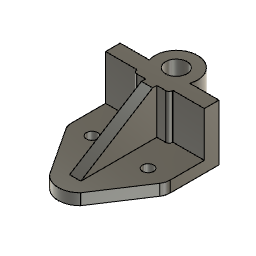
A3 (Autodesk Fusion 360 design; units mm, degrees)
Autodesk Fusion 360 part; units mm, degrees
sketch "Sketch1" plane through (0, 0, 0) normal (0, 0, 1) x (1, 0, 0)
  line L0 (44, 40) -> (-44, 40)
  line L1 (-44, 40) -> (-44, -40)
  line L2 (44, -40) -> (44, 40)
  circle A0 centre (25, -4) radius 5
  circle A1 centre (-25, -4) radius 5
  arc A2 (-13.8302, -53.0279) -> (13.8302, -53.0279) centre (0, -40) ccw
  line L3 (-44, -40) -> (-13.8302, -53.0279)
  line L4 (13.8302, -53.0279) -> (44, -40)
  dimension "d1" = 88
  dimension "d2" = 80
  dimension "d7" = 10
  dimension "d8" = 10
  dimension "d9" = 19
  constraint horizontal L0
  constraint perpendicular L0 L1
  constraint parallel L1 L2
  measures "d1" distance of L1.end L2.start
  measures "d2" distance of L0.end L1.end
  measures "d7" diameter of A0
  measures "d8" diameter of A1
  measures "d9" radius of A2
extrude "Extrude1" add sketch "Sketch1" along normal blind 10
chamfer "Chamfer1" distance 32.8 angle 45 2 edges at (-44, -40, 5) (44, -40, 5)
fillet "Fillet1" radius 13 2 edges at (-44, -7.2, 5) (44, -7.2, 5)
sketch "Sketch2" plane through (0, 0, 0) normal (1, 0, 0) x (0, 1, 0)
  line L0 (40, 10) -> (40, 0) construction
  line L1 (20, 10) -> (20, 50)
  line L2 (20, 10) -> (-44, 10)
  line L3 (20, 50) -> (-44, 10)
  dimension "d15" = 20
  dimension "d16" = 64
  dimension "d17" = 40
  constraint vertical L0
  constraint parallel L0 L1
  constraint perpendicular L1 L2
  measures "d15" distance of L0 L1
  measures "d16" distance of L1.start L2.end
  measures "d17" distance of L1.start L1.end
extrude "Extrude2" add sketch "Sketch2" along normal mid plane 10
sketch "Sketch3" plane through (0, 0, 0) normal (0, 0, 1) x (1, 0, 0)
  line L0 (-44, 40.1) -> (-44, 27.1)
  line L1 (44, 27.1) -> (44, 40.1)
  circle A0 centre (0, 46.1) radius 9.5
  line L2 (5, 23.7404) -> (16, 23.7404)
  line L3 (16, 23.7404) -> (5, 23.7404)
  line L4 (-5, 23.7404) -> (-16, 23.7404)
  line L5 (-16, 23.7404) -> (-16, 27.1)
  line L6 (16, 23.7404) -> (16, 27.1)
  line L7 (5, 20) -> (5, 23.7404)
  line L8 (-5, 20) -> (-5, 23.7404)
  arc A1 (18.0278, 40.1) -> (-18.0278, 40.1) centre (0, 46.1) ccw
  line L9 (-5, 20) -> (5, 20)
  line L10 (44, 40.1) -> (18.0278, 40.1)
  line L11 (-18.0278, 40.1) -> (-44, 40.1)
  line L12 (-44, 27.1) -> (-16, 27.1)
  line L13 (16, 27.1) -> (44, 27.1)
  dimension "d20" = 13
  dimension "d22" = 19
  dimension "d23" = 19
  constraint horizontal L10
  constraint vertical L0
  constraint horizontal L12
  constraint vertical L1
  constraint concentric A0 A1
  constraint perpendicular L1 L2
  constraint parallel L2 L4
  constraint perpendicular L5 L12
  constraint coincident L6.end L12
  constraint perpendicular L6 L12
  constraint perpendicular L3 L7
  constraint perpendicular L4 L8
  constraint coincident A1.end L10
  constraint perpendicular L7 L9
  constraint collinear L10 L11
  constraint collinear L12 L13
  measures "d20" distance of L10 L12
  measures "d22" radius of A1
  measures "d23" diameter of A0
extrude "Extrude3" add sketch "Sketch3" along normal blind 50
fillet "Fillet2" radius 3 2 edges at (-16, 23.7404, 30) (16, 23.7404, 30)
equation "d2 = 67 mm + 13 mm"
